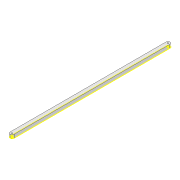
# Autodesk Inventor part: Part_13
Saved by Autodesk Inventor 2022 (Build 260153000, 153)
## iProperties
Created: 2022-04-26
Part Number: Part_13
Material: Generic
Document SubType Name: Modeling
Designer: dell
Density: 1 g/cm^3
Appearance: Default
Author: dell
Autodesk Inventor part; units mm, degrees
ref_plane "YZ Plane" through (0, 0, 0) normal (1, 0, 0) x (0, 1, 0)
ref_plane "XZ Plane" through (0, 0, 0) normal (0, 1, 0) x (-1, 0, 0)
ref_plane "XY Plane" through (0, 0, 0) normal (0, 0, 1) x (1, 0, 0)
sketch "Sketch1" plane through (0, 0, 0) normal (0, 1, 0) x (-1, 0, 0)
  line L0 (0, 0) -> (0, -388.032) construction
  line L1 (-5, 0) -> (-5, -388.032)
  line L2 (5, -388.032) -> (5, 0)
  arc A0 (5, 0) -> (-5, 0) centre (0, 0) ccw
  arc A1 (-5, -388.032) -> (5, -388.032) centre (0, -388.032) ccw
  circle A2 centre (0, 0) radius 1.5
  circle A3 centre (0, -388.032) radius 1.5
  point P0 (0, -194.016)
  dimension "d0" = 388.032
  dimension "d1" = 10
  dimension "d2" = 3
  dimension "d3" = 3
  constraints: 8 end point, 4 centre point, 4 point on circle, 4 tangent, 2 coincident, 1 midpoint, 1 parallel, 1 vertical
  measures "d0" distance of L0.start L0.end
  measures "d1" diameter of A1
  measures "d2" diameter of A2
  measures "d3" diameter of A3
extrude "Extrusion1" add sketch "Sketch1" along normal blind 8
sketch "Sketch2" plane through (0, 0, 0) normal (0, -1, 0) x (1, 0, 0)
  arc A0 (-5, -388.032) -> (5, -388.032) centre (0, -388.032) ccw projected
  line L0 (5, 0) -> (5, -388.032) projected
  arc A1 (5, 0) -> (-5, 0) centre (0, 0) ccw projected
  line L1 (-5, -388.032) -> (-5, 0) projected
  circle A2 centre (0, -388.032) radius 1.5 projected
  circle A3 centre (0, 0) radius 1.5 projected
body "Solid1"
